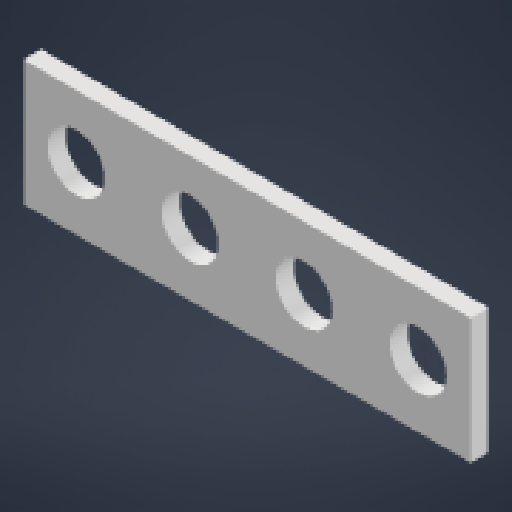
# Autodesk Inventor part: protector_small1x1
Saved by Autodesk Inventor 2024 (Build 280153000, 153)
## iProperties
Created: 2026-04-07
Part Number: protector_small1x1
Material: Generic
Document SubType Name: Modeling
Designer: schar
Density: 1 g/cm^3
Appearance: Default
Author: schar
Autodesk Inventor part; units mm, degrees
ref_plane "YZ Plane" through (0, 0, 0) normal (1, 0, 0) x (0, 1, 0)
ref_plane "XZ Plane" through (0, 0, 0) normal (0, 1, 0) x (-1, 0, 0)
ref_plane "XY Plane" through (0, 0, 0) normal (0, 0, 1) x (1, 0, 0)
sketch "Sketch1" plane through (0, 0, 0) normal (0, 0, 1) x (1, 0, 0)
  circle A0 centre (-19.0795, 0) radius 3.175 projected
  circle A1 centre (-6.3598, 0) radius 3.175 projected
  circle A2 centre (6.3597, 0) radius 3.175 projected
  circle A3 centre (19.0795, 0) radius 3.175 projected
  line L0 (25, -19) -> (25, 19) projected
  line L1 (-25, 19) -> (-25, -19) projected
  line L2 (-19.0795, 0) -> (-6.3598, 0)
  line L3 (-6.3598, 0) -> (-12.7197, 0)
  line L4 (-19.0795, 0) -> (-25.4395, 0)
  line L5 (19.0795, 0) -> (25.4395, 0)
  line L6 (-12.2197, 7) -> (-12.2197, -7)
  line L7 (-12.2197, -7) -> (-13.2197, -7)
  line L8 (-13.2197, -7) -> (-13.2197, 7)
  line L9 (-13.2197, 7) -> (-12.2197, 7)
  line L10 (-12.2197, 7) -> (-13.2197, -7) construction
  line L11 (-12.2197, -7) -> (-13.2197, 7) construction
  line L12 (-25.4395, 0) -> (-25.9395, 0)
  line L13 (-25.9395, 0) -> (-25.9395, 7)
  line L14 (25.4395, 0) -> (25.9395, 0)
  line L15 (25.9395, 0) -> (25.9395, -7)
  line L16 (-25.9395, 7) -> (25.9395, 7)
  line L17 (25.9395, 7) -> (25.9395, -7)
  line L18 (25.9395, -7) -> (-25.9395, -7)
  line L19 (-25.9395, -7) -> (-25.9395, 7)
  point P0 (0, 0)
  point P1 (-25, 7)
  point P2 (-25, -7)
  point P3 (25, -7)
  point P4 (25, 7)
  dimension "d0" = 6.36
  dimension "d1" = 6.36
  dimension "d2" = 14
  dimension "d3" = 1
  dimension "d4" = 0.5
  dimension "d5" = 7
  dimension "d6" = 0.5
  dimension "d7" = 7
  constraints: 36 end point, 5 horizontal, 5 perpendicular, 4 parallel, 3 midpoint, 1 point on line
  measures "d0" distance of L2.start L4.end
  measures "d1" distance of L5.start L5.end
  measures "d2" distance of L6.start L6.end
  measures "d3" distance of L6.end L7.end
  measures "d4" distance of L4.end L12.end
  measures "d5" distance of L12.end L13.end
  measures "d6" distance of L5.end L14.end
  measures "d7" distance of L14.end L15.end
extrude "Extrusion1" add sketch "Sketch1" along normal blind 2 contours L2 L8 L18 L1 L4 A0 | A0 L4 L1 L16 L8 L2 | L8 L9 L6 L2 | L2 L6 L7 L8 | L6 L16 L0 L18
sketch "Sketch2" plane through (0, 0, 2) normal (0, 0, 1) x (1, 0, 0)
  line L0 (-25, 7) -> (-25, -7) projected
  line L1 (-25, 7) -> (-24, 7)
  line L2 (25, 7) -> (-25, 7) projected
  circle A0 centre (-19.0795, 0) radius 3.175 projected
  circle A1 centre (-6.3598, 0) radius 3.175 projected
  line L3 (-19.0795, 0) -> (-6.3598, 0)
  line L4 (-13.2197, 7) -> (-13.2197, -7)
  line L5 (-13.2197, -7) -> (-12.2197, -7)
  line L6 (-12.2197, -7) -> (-12.2197, 7)
  line L7 (-12.2197, 7) -> (-13.2197, 7)
  line L8 (-13.2197, 7) -> (-12.2197, -7) construction
  line L9 (-13.2197, -7) -> (-12.2197, 7) construction
  line L10 (-0.5, 7) -> (-0.5, -7)
  line L11 (-0.5, -7) -> (0.5, -7)
  line L12 (0.5, -7) -> (0.5, 7)
  line L13 (0.5, 7) -> (-0.5, 7)
  line L14 (-0.5, 7) -> (0.5, -7) construction
  line L15 (-0.5, -7) -> (0.5, 7) construction
  circle A2 centre (6.3597, 0) radius 3.175 projected
  circle A3 centre (19.0795, 0) radius 3.175 projected
  line L16 (6.3597, 0) -> (19.0795, 0)
  line L17 (12.2196, 7) -> (12.2196, -7)
  line L18 (12.2196, -7) -> (13.2196, -7)
  line L19 (13.2196, -7) -> (13.2196, 7)
  line L20 (13.2196, 7) -> (12.2196, 7)
  line L21 (12.2196, 7) -> (13.2196, -7) construction
  line L22 (12.2196, -7) -> (13.2196, 7) construction
  line L23 (-24, 7) -> (-25, 7)
  line L24 (-25, 7) -> (-25, -7)
  line L25 (-25, -7) -> (-24, -7)
  line L26 (-24, -7) -> (-24, 7)
  line L27 (25, -7) -> (25, 7) projected
  line L28 (-25, -7) -> (25, -7) projected
  line L29 (25, 7) -> (24, 7)
  line L30 (24, 7) -> (24, -7)
  line L31 (24, -7) -> (25, -7)
  line L32 (25, -7) -> (25, 7)
  point P0 (0, 0)
  point P1 (-12.7197, 0)
  point P2 (12.7196, 0)
  dimension "d10" = 1
  dimension "d11" = 1
  dimension "d12" = 1
  dimension "d13" = 1
  dimension "d14" = 1
  constraints: 58 end point, 10 parallel, 8 midpoint, 7 perpendicular, 4 horizontal, 1 point on line, 2 other
  measures "d10" distance of L0.start L1.end
  measures "d11" distance of L5.end L4.end
  measures "d12" distance of L11.end L10.end
  measures "d13" distance of L18.end L17.end
  measures "d14" distance of L31.end L30.end
extrude "Extrusion2" add sketch "Sketch2" along normal blind 15 contours L1 L26 L25 L0 | L2 L6 L3 L4 | L4 L3 L6 L5 | L2 L12 L11 L10 | L2 L19 L16 L17 | L17 L16 L19 L18 | L2 L27 L28 L30
sketch "Sketch3" plane through (-25, -7, 0) normal (-1, 0, 0) x (0, 0, 1)
  line L0 (2, 14) -> (2, 0) projected
  line L1 (0, 14) -> (17, 14) projected
  line L2 (0, 0) -> (17, 0) projected
  line L3 (14, 14) -> (3, 14)
  line L4 (3, 14) -> (3, 0)
  line L5 (3, 0) -> (14, 0)
  line L6 (17, 3) -> (17, 11)
  line L7 (7.5, 11.5) -> (12.5, 11.5)
  line L8 (14.5, 9.5) -> (14.5, 4.5)
  line L9 (12.5, 2.5) -> (7.5, 2.5)
  line L10 (5.5, 4.5) -> (5.5, 9.5)
  line L11 (5.5, 11.5) -> (14.5, 2.5) construction
  line L12 (14.5, 11.5) -> (5.5, 2.5) construction
  arc A0 (17, 11) -> (14, 14) centre (14, 11) ccw
  arc A1 (14, 0) -> (17, 3) centre (14, 3) ccw
  arc A2 (14.5, 9.5) -> (12.5, 11.5) centre (12.5, 9.5) ccw
  arc A3 (12.5, 2.5) -> (14.5, 4.5) centre (12.5, 4.5) ccw
  arc A4 (7.5, 11.5) -> (5.5, 9.5) centre (7.5, 9.5) ccw
  arc A5 (5.5, 4.5) -> (7.5, 2.5) centre (7.5, 4.5) ccw
  line L13 (17, 14) -> (17, 0) projected
  line L14 (0, 14) -> (17, 14) projected
  point P0 (0, 7)
  point P1 (10, 7)
  dimension "d18" = 14
  dimension "d19" = 9
  dimension "d20" = 9
  dimension "d21" = 3
  dimension "d22" = 3
  dimension "d23" = 2
  constraints: 20 end point, 13 point on line, 12 point on circle, 12 tangent, 6 centre point, 4 parallel, 3 equal radius, 2 horizontal, 2 midpoint, 2 perpendicular
  measures "d18" distance of point (17, 0) L4.end
  measures "d19" distance of L11.end L12.end
  measures "d20" distance of L12.start L11.end
  measures "d21" radius of A0
  measures "d22" radius of A1
  measures "d23" radius of A2
extrude "Extrusion3" cut sketch "Sketch3" against normal through all contours L1 L13 A0 | A1 L13 L2 | L7 A2 L8 A3 L9 A5 L10 A4
body "Solid1"
